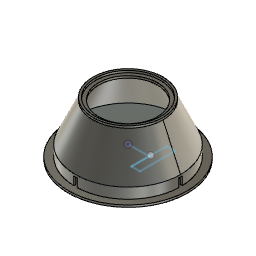
device_modeling v2 (Autodesk Fusion 360 design; units mm, degrees)
Autodesk Fusion 360 part; units mm, degrees
note: some values were not read from the file. Set by a fixed rule: which sketch regions a step uses.
sketch "bottom" plane through (0, 0, 0) normal (0, 1, 0) x (1, 0, 0)
  line L0 (0, 0) -> (85, 0)
  line L1 (85, 0) -> (85, -3)
  line L2 (85, -3) -> (0, -3)
  line L3 (0, -3) -> (0, 0)
  dimension "d1" = 3
  dimension "d2" = 85
  constraint horizontal L0
  constraint vertical L1
  constraint horizontal L2
  constraint vertical L3
  constraint coincident L0.start L3.end
  measures "d1" distance of L0.end L1.end
  measures "d2" distance of L0.start L0.end
revolve "Revolve3" add sketch "bottom" angle 360 about axis through (0, 0, 1.75) along (0, 0, 1) makes body 1
sketch "center" plane through (0, 0, 0) normal (0, 1, 0) x (1, 0, 0)
  line L0 (85, -3) -> (72, -3)
  line L1 (72, -3) -> (75, -3)
  line L2 (75, -3) -> (75, -18)
  line L3 (75, -18) -> (72, -18)
  line L4 (72, -18) -> (72, -3)
  line L5 (72, -18) -> (0, -18)
  line L6 (0, -18) -> (0, -15)
  line L7 (0, -15) -> (72, -15)
  line L8 (72, -15) -> (72, -18)
  dimension "d3" = 13
  dimension "d4" = 15
  dimension "d5" = 3
  dimension "d6" = 72
  dimension "d7" = 3
  constraint horizontal L0
  constraint horizontal L1
  constraint vertical L2
  constraint horizontal L3
  constraint vertical L4
  constraint horizontal L5
  constraint vertical L6
  constraint horizontal L7
  constraint vertical L8
  measures "d3" distance of L0.start L0.end
  measures "d4" distance of L1.end L2.end
  measures "d5" distance of L0.end L1.end
  measures "d6" distance of L3.end L5.end
  measures "d7" distance of L3.end L7.end
sketch "top" plane through (0, 0, 0) normal (0, 1, 0) x (1, 0, 0)
  line L0 (50, -76) -> (47, -76)
  line L1 (47, -76) -> (47, -73)
  line L2 (47, -73) -> (50, -73)
  line L3 (50, -73) -> (50, -76)
  line L4 (50, -73) -> (42, -73)
  line L5 (42, -73) -> (42, -70)
  line L6 (47, -76) -> (42, -76)
  line L7 (47, -73) -> (47, -70)
  line L8 (42, -73) -> (0, -73)
  line L9 (42, -70) -> (47, -70)
  line L10 (0, 0) -> (0, -18)
  line L11 (0, -18) -> (72, -18)
  line L12 (72, -18) -> (75, -18)
  spline S0 degree 5 poles (47, -70) (48, -67.92) (50, -63.76) (53, -57.52) (57, -49.2) (62, -38.8) (66, -30.48) (69, -24.24) (71, -20.08) (72, -18) knots 0 0 0 0 0 0 0.2 0.4 0.6 0.8 1 1 1 1 1 1
  spline S1 degree 5 poles (50, -73) (51, -70.8) (53, -66.4) (56, -59.8) (60, -51) (65, -40) (69, -31.2) (72, -24.6) (74, -20.2) (75, -18) knots 0 0 0 0 0 0 0.2 0.4 0.6 0.8 1 1 1 1 1 1
  dimension "d10" = 3
  dimension "d11" = 3
  dimension "d12" = 8
  dimension "d13" = 3
  dimension "d14" = 5
  dimension "d20" = 42
  dimension "d23" = 18
  dimension "d25" = 72
  dimension "d26" = 3
  constraint horizontal L0
  constraint vertical L1
  constraint horizontal L2
  constraint vertical L3
  constraint horizontal L4
  constraint vertical L5
  constraint perpendicular L7 L9
  constraint coincident L10.start origin
  constraint vertical L10
  constraint perpendicular L10 L11
  constraint horizontal L12
  constraint coincident L2.end L3.start
  measures "d10" distance of L0.start L0.end
  measures "d11" distance of L0.start L2.end
  measures "d12" distance of L2.end L4.end
  measures "d13" distance of L4.end L5.end
  measures "d14" distance of L0.end L6.end
  measures "d20" distance of L4.end L8.end
  measures "d23" distance of L10.start L10.end
  measures "d25" distance of L10.end L11.end
  measures "d26" distance of L11.end L12.end
revolve "Revolve4" add sketch "center" angle 360 about axis through (0, 0, 1.75) along (0, 0, 1) separate body makes body 2
revolve "Revolve5" add sketch "top" angle 360 about axis through (0, 0, 1.75) along (0, 0, 1) separate body makes body 3
sketch "bottom hole" plane through (0, 0, 0) normal (0, 0, 1) x (1, 0, 0)
  line L0 (0, 0) -> (40, 0)
  line L1 (40, 0) -> (40, -40)
  line L2 (40, -40) -> (-40, -40)
  line L3 (-40, -40) -> (-40, 40)
  line L4 (-40, 40) -> (40, 40)
  line L5 (40, 40) -> (40, -40)
  dimension "d32" = 40
  dimension "d33" = 40
  dimension "d34" = 80
  dimension "d35" = 80
  constraint coincident L0.start origin
  constraint horizontal L0
  constraint perpendicular L0 L1
  constraint horizontal L2
  constraint vertical L3
  constraint horizontal L4
  constraint vertical L5
  measures "d32" distance of L0.start L0.end
  measures "d33" distance of L0.end L1.end
  measures "d34" distance of L1.end L2.end
  measures "d35" distance of L1.end L4.end
extrude "Extrude1" cut sketch "bottom hole" along normal blind 3 bodies 1
sketch "center_ center hole" plane through (0, 0, 18) normal (0, 0, 1) x (-1, 0, 0)
  circle A0 centre (0, 0) radius 75
  line L0 (0, 0) -> (-30, 0)
  line L1 (-30, 0) -> (-30, 25)
  line L2 (-30, 25) -> (-42, 25)
  line L3 (-42, 25) -> (-42, -25)
  line L4 (-42, -25) -> (-30, -25)
  line L5 (-30, -25) -> (-30, 25)
  line L6 (-30, -2.5) -> (-30, 0)
  dimension "d39" = 30
  dimension "d40" = 25
  dimension "d41" = 12
  dimension "d42" = 50
  constraint coincident A0.centre L0.start
  constraint horizontal L2
  constraint vertical L3
  constraint horizontal L4
  constraint vertical L5
  constraint vertical L6
  measures "d39" distance of A0.centre L0.end
  measures "d40" distance of L0.end L1.end
  measures "d41" distance of L1.end L2.end
  measures "d42" distance of L1.end L4.end
extrude "Extrude8" cut sketch "center_ center hole" against normal blind 3 contours L1 L2 L3 L4 L5 L6 bodies 2
sketch "Sketch10" plane through (0, 0, 15) normal (0, 0, -1) x (1, 0, 0)
  circle A0 centre (0, 0) radius 72
  line L0 (0, 0) -> (0, -2.5)
  line L1 (0, -2.5) -> (0, 2.5)
  line L2 (0, 2.5) -> (-102.7298, 2.5)
  line L3 (-102.7298, 2.5) -> (128.2969, 2.5)
  line L4 (-102.7298, 2.5) -> (93.6232, 2.5)
  line L5 (93.6232, 2.5) -> (93.6232, -2.5)
  line L6 (93.6232, -2.5) -> (-102.7298, -2.5)
  line L7 (-102.7298, -2.5) -> (-102.7298, 2.5)
  line L8 (30, 25) -> (42, 25)
  line L9 (42, 25) -> (42, -25)
  line L10 (42, -25) -> (30, -25)
  line L11 (30, -25) -> (30, 25)
  dimension "d50" = 5
  dimension "d51" = 2.5
  dimension "d52" = 5
  constraint coincident A0.centre L0.start
  constraint vertical L0
  constraint parallel L0 L1
  constraint perpendicular L1 L2
  constraint perpendicular L1 L3
  constraint horizontal L4
  constraint vertical L5
  constraint horizontal L6
  constraint vertical L7
  measures "d50" distance of L0.end L1.end
  measures "d51" distance of A0.centre L0.end
  measures "d52" distance of L2.end L6.end
extrude "Extrude5" cut sketch "Sketch10" along normal blind 12 contours A0 L3 L4 L5 L6 bodies 2
extrude "Extrude4" cut sketch "Sketch10" along normal blind 12 contours A0 L2 L3 L4 L6 L7 bodies 2
sketch "Sketch11" plane through (0, 0, 15) normal (0, 0, -1) x (1, 0, 0)
  line L0 (0, 0) -> (2.5, 0)
  line L1 (2.5, 0) -> (-2.5, 0)
  line L2 (-2.5, 0) -> (2.5, 0)
  line L3 (2.5, 0) -> (2.5, 75)
  line L4 (2.5, 75) -> (-2.5, 75)
  line L5 (-2.5, 75) -> (-2.5, 0)
  line L6 (2.5, 0) -> (-2.5, 0)
  line L7 (-2.5, 0) -> (-2.5, -75)
  line L8 (-2.5, -75) -> (2.5, -75)
  line L9 (2.5, -75) -> (2.5, 0)
  dimension "d57" = 5
  dimension "d58" = 2.5
  dimension "d59" = 5
  dimension "d60" = 75
  dimension "d61" = 75
  dimension "d62" = 5
  constraint coincident L0.start origin
  constraint horizontal L0
  constraint parallel L0 L1
  constraint horizontal L2
  constraint vertical L3
  constraint horizontal L4
  constraint vertical L5
  constraint horizontal L6
  constraint vertical L7
  constraint horizontal L8
  constraint vertical L9
  measures "d57" distance of L0.end L1.end
  measures "d58" distance of L0.start L0.end
  measures "d59" distance of L1.end L0.end
  measures "d60" distance of L1.end L4.end
  measures "d61" distance of L0.end L8.end
  measures "d62" distance of L7.end L8.end
extrude "Extrude7" cut sketch "Sketch11" along normal blind 12 contours L0 L1 L2 L3 L4 L5 L6 bodies 2
extrude "Extrude6" cut sketch "Sketch11" along normal blind 12 contours L0 L1 L2 L6 L7 L8 L9 bodies 2
extrude "Extrude3" cut sketch "center_ center hole" against normal blind 3 contours L1 L2 L3 L4 L5 L6 bodies 2
extrude "Extrude2" cut sketch "center_ center hole" against normal blind 3 contours L1 L2 L3 L4 L5 L6 bodies 2
named bodies: "bottom", "center", "top"
